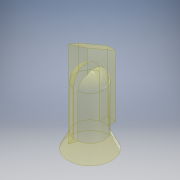
# Autodesk Inventor part: Cutter
Saved by Autodesk Inventor 2017 (Build 210142000, 142)
## iProperties
Created: 2021-02-25
Part Number: Cutter
Material: Generic
Document SubType Name: Modeling
Designer: Lenovo Y900
Density: 1 g/cm^3
Appearance: Clear - Yellow
Author: Lenovo Y900
Autodesk Inventor part; units mm, degrees
ref_plane "YZ Plane" through (0, 0, 0) normal (1, 0, 0) x (0, 1, 0)
ref_plane "XZ Plane" through (0, 0, 0) normal (0, 1, 0) x (-1, 0, 0)
ref_plane "XY Plane" through (0, 0, 0) normal (0, 0, 1) x (1, 0, 0)
sketch "Sketch1" plane through (0, 0, 0) normal (0, 0, 1) x (1, 0, 0)
  circle A0 centre (0, 0) radius 7.5
  dimension "d0" = 15
  constraints: 1 centre point, 1 coincident
  measures "d0" diameter of A0
ref_plane "Work Plane1" through (0, 0, 5) normal (0, 0, 1) x (1, 0, 0)
sketch "Sketch2" plane through (0, 0, 5) normal (0, 0, 1) x (1, 0, 0)
  circle A0 centre (0, 0) radius 5
  dimension "d4" = 10
  constraints: 1 centre point, 1 coincident
  measures "d4" diameter of A0
loft "Loft1" add profiles "Sketch1", "Sketch2"
sketch "Sketch3" plane through (0, 0, 5) normal (0, 0, 1) x (1, 0, 0)
  circle A0 centre (0, 0) radius 5
  dimension "d9" = 10
  constraints: 1 centre point, 1 coincident
  measures "d9" diameter of A0
extrude "Extrusion2" add sketch "Sketch3" along normal blind 15
sketch "Sketch4" plane through (0, 0, 20) normal (0, 0, 1) x (1, 0, 0)
  line L0 (5, 0) -> (-5, 0)
  arc A0 (-5, 0) -> (5, 0) centre (0, 0) ccw
  constraints: 2 end point, 2 point on circle, 1 centre point, 1 horizontal
revolve "Revolution1" add sketch "Sketch4" angle 180 about axis through (5, 0, 20) along (-1, 0, 0)
ref_plane "Work Plane2" through (0, 0, 5) normal (0, 0, -1) x (-1, 0, 0)
sketch "Sketch6" plane through (0, 0, 5) normal (0, 0, -1) x (-1, 0, 0)
  line L0 (-1.5, 7.5) -> (1.5, 7.5)
  line L1 (1.5, -2.5) -> (0, -7.5)
  line L2 (0, -7.5) -> (-1.5, -2.5)
  line L3 (1.5, 7.5) -> (1.5, -2.5)
  line L4 (-1.5, -2.5) -> (-1.5, 7.5)
  line L5 (0.9, -4.5) -> (-1.5, 7.5) construction
  line L6 (-0.9, -4.5) -> (1.5, 7.5) construction
  point P0 (0, 0)
  point P1 (0, 7.5)
  point P2 (0, 0)
  dimension "d14" = 3
  constraints: 14 end point, 4 point on line, 1 parallel
  measures "d14" distance of L0.start L0.end
extrude "Extrusion3" add sketch "Sketch6" against normal blind 30
ref_plane "Work Plane3" through (1.5, 7.5, 35) normal (0, 0.5, 0.8660254) x (-1, 0, 0)
sketch "Sketch7" plane through (1.5, 7.5, 35) normal (0, 0.5, 0.8660254) x (-1, 0, 0)
  line L0 (0, 16.105) -> (3, 16.105)
  line L1 (3, 16.105) -> (3, -7.3572)
  line L2 (3, -7.3572) -> (0, -7.3572)
  line L3 (0, -7.3572) -> (0, 16.105)
  line L4 (0, 16.105) -> (3, -7.3572) construction
  line L5 (3, 16.105) -> (0, -7.3572) construction
  point P0 (1.5, -11.0048)
  point P1 (1.5, 4.3739)
  dimension "d19" = 23.4622
  constraints: 12 end point, 2 midpoint, 2 parallel, 1 horizontal, 1 perpendicular
  measures "d19" distance of L0.end L1.end
extrude "Extrusion4" cut sketch "Sketch7" against normal blind 7.5
body "Solid2"
